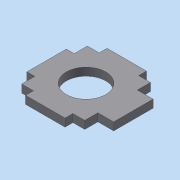
# Autodesk Inventor part: Y-Anchor_Bearing-Ring-Middle
Saved by Autodesk Inventor 2016 SP1 (Build 200210100, 210)
## iProperties
Created: 2016-01-20
Part Number: Y-Anchor_Bearing-Ring-Middle
Material: Generic
Document SubType Name: Modeling
Designer: Mohamed A.
Density: 1 g/cm^3
Appearance: Default
Author: Mohamed A.
Autodesk Inventor part; units mm, degrees
ref_plane "YZ Plane" through (0, 0, 0) normal (1, 0, 0) x (0, 1, 0)
ref_plane "XZ Plane" through (0, 0, 0) normal (0, 1, 0) x (-1, 0, 0)
ref_plane "XY Plane" through (0, 0, 0) normal (0, 0, 1) x (1, 0, 0)
sketch "Sketch1" plane through (0, 0, 0) normal (0, 0, 1) x (1, 0, 0)
  circle A0 centre (0, 0) radius 7.5
  line L0 (15.0015, 7.5) -> (12.0015, 7.5)
  line L1 (12.0015, 7.5) -> (12.0015, 12.5)
  line L2 (12.0015, -12.5) -> (12.0015, -7.5)
  line L3 (12.0015, -7.5) -> (15.0015, -7.5)
  line L4 (-7.5, -15.5) -> (-7.5, -12.5)
  line L5 (-7.5, -12.5) -> (-12, -12.5)
  line L6 (7.5, -15.5) -> (7.5, -12.5)
  line L7 (7.5, -12.5) -> (12.0015, -12.5)
  line L8 (-15, -7.5) -> (-12, -7.5)
  line L9 (-12, -7.5) -> (-12, -12.5)
  line L10 (-15, 7.5) -> (-12, 7.5)
  line L11 (-12, 7.5) -> (-12, 12.5)
  line L12 (-7.5, 15.5) -> (-7.5, 12.5)
  line L13 (-7.5, 12.5) -> (-12, 12.5)
  line L14 (12.0015, 12.5) -> (7.5, 12.5)
  line L15 (7.5, 12.5) -> (7.5, 15.5)
  line L16 (15.0015, 7.5) -> (15.0015, -7.5)
  line L17 (-7.5, 15.5) -> (7.5, 15.5)
  line L18 (-15, -7.5) -> (-15, 7.5)
  line L19 (7.5, -15.5) -> (-7.5, -15.5)
  line L20 (15.0015, 7.5) -> (18.0015, 7.5)
  line L21 (18.0015, 7.5) -> (18.0015, -7.5)
  line L22 (18.0015, -7.5) -> (15.0015, -7.5)
  line L23 (15.0015, -7.5) -> (15.0015, 7.5)
  line L24 (-20.9424, 0) -> (31.3224, 0) construction
  dimension "d0" = 15
  dimension "d3" = 3
  dimension "d5" = 3
  dimension "d6" = 3
  dimension "d7" = 15
  dimension "d9" = 15
  dimension "d13" = 3
  dimension "d15" = 31
  dimension "d16" = 3
  constraints: 50 end point, 12 point on line, 9 perpendicular, 5 horizontal, 4 parallel, 2 collinear, 1 centre point, 1 coincident, 1 other
  measures "d0" diameter of A0
  measures "d3" distance of L0.start L0.end
  measures "d5" distance of L8.start L8.end
  measures "d6" distance of L12.start L12.end
  measures "d7" distance between parallel lines of L3 L0
  measures "d9" distance between parallel lines of L12 L15
  measures "d13" distance of L21.end L22.end
  measures "d15" distance between parallel lines of L19 L17
  measures "d16" distance of L6.start L6.end
extrude "Extrusion1" add sketch "Sketch1" along normal blind 3
body "Solid1"
